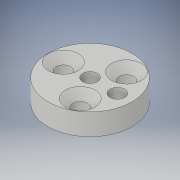
# Autodesk Inventor part: PrzejsciowkaDoFormy
Saved by Autodesk Inventor 2019 (Build 230136000, 136)
## iProperties
Created: 2021-11-09
Part Number: PrzejsciowkaDoFormy
Material: Ogólny
Document SubType Name: Modeling
Designer: Michał
Density: 1 g/cm^3
Appearance: Domyślna
Author: Michał
Autodesk Inventor part; units mm, degrees
ref_plane "YZ Plane" through (0, 0, 0) normal (1, 0, 0) x (0, 1, 0)
ref_plane "XZ Plane" through (0, 0, 0) normal (0, 1, 0) x (-1, 0, 0)
ref_plane "XY Plane" through (0, 0, 0) normal (0, 0, 1) x (1, 0, 0)
sketch "Szkic1" plane through (0, 0, 0) normal (0, 1, 0) x (-1, 0, 0)
  circle A0 centre (0, 0) radius 9.75
  dimension "d0" = 19.5
  constraints: 1 centre point, 1 coincident
  measures "d0" diameter of A0
extrude "Wyciągnięcie proste1" add sketch "Szkic1" along normal blind 5
sketch "Szkic2" plane through (0, 5, 0) normal (0, 1, 0) x (1, 0, 0)
  line L0 (0, 0) -> (-6.2, 0) construction
  line L1 (0, 0) -> (3.1, 5.3694) construction
  line L2 (0, 0) -> (3.1, -5.3694) construction
  dimension "d3" = 6.2
  dimension "d4" = 120
  dimension "d5" = 120
  constraints: 6 end point, 3 coincident, 2 equal length, 1 horizontal
  measures "d3" distance of L0.start L0.end
  measures "d4" angle of L0 L1
  measures "d5" angle of L1 L2
hole "Otwór1" at (-6.2, 5, 0) at (3.1, 5, -5.3694) at (3.1, 5, 5.3694) direction (0, -1, 0) diameter 3.4 end through all countersink diameter 6.9 countersink angle 89.954 clearance for "Śruba ze łbem stożkowym ISO 2009/7046" size "M3" standard "ISO"
sketch "Szkic3" plane through (0, 5, 0) normal (0, 1, 0) x (1, 0, 0)
  line L0 (0, 0) -> (6.35, 0)
  dimension "d13" = 6.35
  constraints: 2 end point, 1 horizontal
  measures "d13" distance of L0.start L0.end
hole "Otwór2" at (0, 5, 0) at (6.35, 5, 0) direction (0, -1, 0) diameter 3.4 end through all
